Autodesk Fusion 360 part; units mm, degrees
(part 6 of 9)
sketch "草图17 (8)" plane through (593, 0, 0) normal (1, 0, 0) x (0, 0, -1) in component "R1_DrainPan"
  line L0 (-24.9649, 136.9) -> (-24.6782, 141)
  line L1 (-24.6782, 141) -> (-41, 141)
  line L2 (-41, 141) -> (-41, 136.9)
  line L3 (-41, 136.9) -> (-24.9649, 136.9)
  dimension "d2420" = 24.9649
  dimension "d2421" = 136.9
  dimension "d2422" = 24.6782
  dimension "d2423" = 141
  dimension "d2424" = 41
  constraint horizontal L1
  constraint vertical L2
  constraint horizontal L3
  measures "d2420" horizontal distance of origin L0.start
  measures "d2421" vertical distance of origin L0.start
  measures "d2422" horizontal distance of origin L0.end
  measures "d2423" vertical distance of origin L0.end
  measures "d2424" horizontal distance of origin L1.end
extrude "R02 full width open front''" cut sketch "草图17 (8)" along normal blind 128 bodies 13 in component "R1_DrainPan"
ref_plane "工作平面14" through (0, 0, 36) normal (0, 0, 1) x (1, 0, 0) in component "R1_RemovableGrate"
sketch "草图14 (13)" plane through (0, 0, 36) normal (0, 0, 1) x (1, 0, 0) in component "R1_RemovableGrate"
  line L0 (592.7, 59.7) -> (595.3, 59.7)
  line L1 (595.3, 59.7) -> (595.3, 65.3)
  line L2 (595.3, 65.3) -> (592.7, 65.3)
  line L3 (592.7, 65.3) -> (592.7, 59.7)
  dimension "d2430" = 59.7
  dimension "d2431" = 2.6
  dimension "d2432" = 5.6
  constraint horizontal L0
  constraint vertical L1
  constraint horizontal L2
  constraint vertical L3
  measures "d2430" vertical distance of origin L0.start
  measures "d2431" horizontal distance of L0.start L0.end
  measures "d2432" vertical distance of L0.end L1.end
extrude "R02 side locating notch 0''" cut sketch "草图14 (13)" along normal blind 4 bodies 14 in component "R1_RemovableGrate"
ref_plane "工作平面18" through (0, 0, 20) normal (0, 0, 1) x (1, 0, 0) in component "R1_DrainPan"
sketch "草图18 (4)" plane through (0, 0, 20) normal (0, 0, 1) x (1, 0, 0) in component "R1_DrainPan"
  line L0 (593, 60) -> (595, 60)
  line L1 (595, 60) -> (595, 65)
  line L2 (595, 65) -> (593, 65)
  line L3 (593, 65) -> (593, 60)
  dimension "d2438" = 60
  dimension "d2439" = 2
  dimension "d2440" = 5
  constraint horizontal L0
  constraint vertical L1
  constraint horizontal L2
  constraint vertical L3
  measures "d2438" vertical distance of origin L0.start
  measures "d2439" horizontal distance of L0.start L0.end
  measures "d2440" vertical distance of L0.end L1.end
extrude "R02 side locating key 0''" add sketch "草图18 (4)" along normal blind 20 bodies 13 in component "R1_DrainPan"
ref_plane "工作平面15" through (0, 0, 36) normal (0, 0, 1) x (1, 0, 0) in component "R1_RemovableGrate"
sketch "草图15 (13)" plane through (0, 0, 36) normal (0, 0, 1) x (1, 0, 0) in component "R1_RemovableGrate"
  line L0 (718.7, 59.7) -> (721.3, 59.7)
  line L1 (721.3, 59.7) -> (721.3, 65.3)
  line L2 (721.3, 65.3) -> (718.7, 65.3)
  line L3 (718.7, 65.3) -> (718.7, 59.7)
  dimension "d2445" = 718.7
  dimension "d2446" = 59.7
  dimension "d2447" = 2.6
  dimension "d2448" = 5.6
  constraint horizontal L0
  constraint vertical L1
  constraint horizontal L2
  constraint vertical L3
  measures "d2445" horizontal distance of origin L0.start
  measures "d2446" vertical distance of origin L0.start
  measures "d2447" horizontal distance of L0.start L0.end
  measures "d2448" vertical distance of L0.end L1.end
extrude "R02 side locating notch 1''" cut sketch "草图15 (13)" along normal blind 4 bodies 14 in component "R1_RemovableGrate"
ref_plane "工作平面19" through (0, 0, 20) normal (0, 0, 1) x (1, 0, 0) in component "R1_DrainPan"
sketch "草图19 (4)" plane through (0, 0, 20) normal (0, 0, 1) x (1, 0, 0) in component "R1_DrainPan"
  line L0 (719, 60) -> (721, 60)
  line L1 (721, 60) -> (721, 65)
  line L2 (721, 65) -> (719, 65)
  line L3 (719, 65) -> (719, 60)
  dimension "d2453" = 719
  dimension "d2454" = 60
  dimension "d2455" = 2
  dimension "d2456" = 5
  constraint horizontal L0
  constraint vertical L1
  constraint horizontal L2
  constraint vertical L3
  measures "d2453" horizontal distance of origin L0.start
  measures "d2454" vertical distance of origin L0.start
  measures "d2455" horizontal distance of L0.start L0.end
  measures "d2456" vertical distance of L0.end L1.end
extrude "R02 side locating key 1''" add sketch "草图19 (4)" along normal blind 20 bodies 13 in component "R1_DrainPan"
ref_plane "工作平面16" through (0, 0, 19.8) normal (0, 0, 1) x (1, 0, 0) in component "R2_DrainPan"
sketch "草图16 (9)" plane through (0, 0, 19.8) normal (0, 0, 1) x (1, 0, 0) in component "R2_DrainPan"
  line L0 (725, 140) -> (861, 140)
  line L1 (861, 140) -> (861, 167)
  line L2 (861, 167) -> (725, 167)
  line L3 (725, 167) -> (725, 140)
  dimension "d2461" = 725
  dimension "d2463" = 136
  dimension "d2464" = 27
  constraint horizontal L0
  constraint vertical L1
  constraint horizontal L2
  constraint vertical L3
  measures "d2461" horizontal distance of origin L0.start
  measures "d2463" horizontal distance of L0.start L0.end
  measures "d2464" vertical distance of L0.end L1.end
extrude "R02 remove projecting spout'''" cut sketch "草图16 (9)" along normal blind 20.4 bodies 19 in component "R2_DrainPan"
ref_plane "工作平面17" through (729, 0, 0) normal (1, 0, 0) x (0, 1, 0) in component "R2_DrainPan"
sketch "草图17 (9)" plane through (729, 0, 0) normal (1, 0, 0) x (0, 0, -1) in component "R2_DrainPan"
  line L0 (-24.9649, 136.9) -> (-24.6782, 141)
  line L1 (-24.6782, 141) -> (-41, 141)
  line L2 (-41, 141) -> (-41, 136.9)
  line L3 (-41, 136.9) -> (-24.9649, 136.9)
  dimension "d2469" = 24.9649
  dimension "d2470" = 136.9
  dimension "d2471" = 24.6782
  dimension "d2472" = 141
  dimension "d2473" = 41
  constraint horizontal L1
  constraint vertical L2
  constraint horizontal L3
  measures "d2469" horizontal distance of origin L0.start
  measures "d2470" vertical distance of origin L0.start
  measures "d2471" horizontal distance of origin L0.end
  measures "d2472" vertical distance of origin L0.end
  measures "d2473" horizontal distance of origin L1.end
extrude "R02 full width open front'''" cut sketch "草图17 (9)" along normal blind 128 bodies 19 in component "R2_DrainPan"
ref_plane "工作平面14" through (0, 0, 36) normal (0, 0, 1) x (1, 0, 0) in component "R2_RemovableGrate"
sketch "草图14 (14)" plane through (0, 0, 36) normal (0, 0, 1) x (1, 0, 0) in component "R2_RemovableGrate"
  line L0 (728.7, 59.7) -> (731.3, 59.7)
  line L1 (731.3, 59.7) -> (731.3, 65.3)
  line L2 (731.3, 65.3) -> (728.7, 65.3)
  line L3 (728.7, 65.3) -> (728.7, 59.7)
  dimension "d2478" = 728.7
  dimension "d2479" = 59.7
  dimension "d2480" = 2.6
  dimension "d2481" = 5.6
  constraint horizontal L0
  constraint vertical L1
  constraint horizontal L2
  constraint vertical L3
  measures "d2478" horizontal distance of origin L0.start
  measures "d2479" vertical distance of origin L0.start
  measures "d2480" horizontal distance of L0.start L0.end
  measures "d2481" vertical distance of L0.end L1.end
extrude "R02 side locating notch 0'''" cut sketch "草图14 (14)" along normal blind 4 bodies 20 in component "R2_RemovableGrate"
ref_plane "工作平面18" through (0, 0, 20) normal (0, 0, 1) x (1, 0, 0) in component "R2_DrainPan"
sketch "草图18 (5)" plane through (0, 0, 20) normal (0, 0, 1) x (1, 0, 0) in component "R2_DrainPan"
  line L0 (729, 60) -> (731, 60)
  line L1 (731, 60) -> (731, 65)
  line L2 (731, 65) -> (729, 65)
  line L3 (729, 65) -> (729, 60)
  dimension "d2486" = 729
  dimension "d2487" = 60
  dimension "d2488" = 2
  dimension "d2489" = 5
  constraint horizontal L0
  constraint vertical L1
  constraint horizontal L2
  constraint vertical L3
  measures "d2486" horizontal distance of origin L0.start
  measures "d2487" vertical distance of origin L0.start
  measures "d2488" horizontal distance of L0.start L0.end
  measures "d2489" vertical distance of L0.end L1.end
extrude "R02 side locating key 0'''" add sketch "草图18 (5)" along normal blind 20 bodies 19 in component "R2_DrainPan"
ref_plane "工作平面15" through (0, 0, 36) normal (0, 0, 1) x (1, 0, 0) in component "R2_RemovableGrate"
sketch "草图15 (14)" plane through (0, 0, 36) normal (0, 0, 1) x (1, 0, 0) in component "R2_RemovableGrate"
  line L0 (854.7, 59.7) -> (857.3, 59.7)
  line L1 (857.3, 59.7) -> (857.3, 65.3)
  line L2 (857.3, 65.3) -> (854.7, 65.3)
  line L3 (854.7, 65.3) -> (854.7, 59.7)
  dimension "d2494" = 854.7
  dimension "d2495" = 59.7
  dimension "d2496" = 2.6
  dimension "d2497" = 5.6
  constraint horizontal L0
  constraint vertical L1
  constraint horizontal L2
  constraint vertical L3
  measures "d2494" horizontal distance of origin L0.start
  measures "d2495" vertical distance of origin L0.start
  measures "d2496" horizontal distance of L0.start L0.end
  measures "d2497" vertical distance of L0.end L1.end
extrude "R02 side locating notch 1'''" cut sketch "草图15 (14)" along normal blind 4 bodies 20 in component "R2_RemovableGrate"
ref_plane "工作平面19" through (0, 0, 20) normal (0, 0, 1) x (1, 0, 0) in component "R2_DrainPan"
sketch "草图19 (5)" plane through (0, 0, 20) normal (0, 0, 1) x (1, 0, 0) in component "R2_DrainPan"
  line L0 (855, 60) -> (857, 60)
  line L1 (857, 60) -> (857, 65)
  line L2 (857, 65) -> (855, 65)
  line L3 (855, 65) -> (855, 60)
  dimension "d2502" = 855
  dimension "d2503" = 60
  dimension "d2504" = 2
  dimension "d2505" = 5
  constraint horizontal L0
  constraint vertical L1
  constraint horizontal L2
  constraint vertical L3
  measures "d2502" horizontal distance of origin L0.start
  measures "d2503" vertical distance of origin L0.start
  measures "d2504" horizontal distance of L0.start L0.end
  measures "d2505" vertical distance of L0.end L1.end
extrude "R02 side locating key 1'''" add sketch "草图19 (5)" along normal blind 20 bodies 19 in component "R2_DrainPan"
ref_plane "工作平面16" through (0, 0, 19.8) normal (0, 0, 1) x (1, 0, 0) in component "LS_DrainPan"
sketch "草图16 (10)" plane through (0, 0, 19.8) normal (0, 0, 1) x (1, 0, 0) in component "LS_DrainPan"
  line L0 (170, 141) -> (197, 141)
  line L1 (197, 141) -> (197, 323)
  line L2 (197, 323) -> (170, 323)
  line L3 (170, 323) -> (170, 141)
  dimension "d2511" = 141
  dimension "d2512" = 27
  dimension "d2513" = 182
  constraint horizontal L0
  constraint vertical L1
  constraint horizontal L2
  constraint vertical L3
  measures "d2511" vertical distance of origin L0.start
  measures "d2512" horizontal distance of L0.start L0.end
  measures "d2513" vertical distance of L0.end L1.end
extrude "R02 remove projecting spout''''" cut sketch "草图16 (10)" along normal blind 20.4 bodies 25 in component "LS_DrainPan"
ref_plane "工作平面17" through (0, 319, 0) normal (0, 1, 0) x (0, 0, 1) in component "LS_DrainPan"
sketch "草图17 (10)" plane through (0, 319, 0) normal (0, 1, 0) x (1, 0, 0) in component "LS_DrainPan"
  line L0 (166.9, -24.9649) -> (171, -24.6782)
  line L1 (171, -24.6782) -> (171, -41)
  line L2 (171, -41) -> (166.9, -41)
  line L3 (166.9, -41) -> (166.9, -24.9649)
  dimension "d2518" = 166.9
  dimension "d2519" = 24.9649
  dimension "d2520" = 171
  dimension "d2521" = 24.6782
  dimension "d2522" = 41
  constraint vertical L1
  constraint horizontal L2
  constraint vertical L3
  measures "d2518" horizontal distance of origin L0.start
  measures "d2519" vertical distance of origin L0.start
  measures "d2520" horizontal distance of origin L0.end
  measures "d2521" vertical distance of origin L0.end
  measures "d2522" vertical distance of origin L1.end
extrude "R02 full width open front''''" cut sketch "草图17 (10)" against normal blind 174 bodies 25 in component "LS_DrainPan"
ref_plane "工作平面18" through (0, 0, 36) normal (0, 0, 1) x (1, 0, 0) in component "LS_RemovableGrate"
sketch "草图18 (6)" plane through (0, 0, 36) normal (0, 0, 1) x (1, 0, 0) in component "LS_RemovableGrate"
  line L0 (59.7, 316.7) -> (65.3, 316.7)
  line L1 (65.3, 316.7) -> (65.3, 319.3)
  line L2 (65.3, 319.3) -> (59.7, 319.3)
  line L3 (59.7, 319.3) -> (59.7, 316.7)
  dimension "d2527" = 59.7
  dimension "d2528" = 316.7
  dimension "d2529" = 5.6
  dimension "d2530" = 2.6
  constraint horizontal L0
  constraint vertical L1
  constraint horizontal L2
  constraint vertical L3
  measures "d2527" horizontal distance of origin L0.start
  measures "d2528" vertical distance of origin L0.start
  measures "d2529" horizontal distance of L0.start L0.end
  measures "d2530" vertical distance of L0.end L1.end
extrude "R02 side locating notch 0''''" cut sketch "草图18 (6)" along normal blind 4 bodies 26 in component "LS_RemovableGrate"
ref_plane "工作平面18" through (0, 0, 20) normal (0, 0, 1) x (1, 0, 0) in component "LS_DrainPan"
sketch "草图18 (7)" plane through (0, 0, 20) normal (0, 0, 1) x (1, 0, 0) in component "LS_DrainPan"
  line L0 (60, 317) -> (65, 317)
  line L1 (65, 317) -> (65, 319)
  line L2 (65, 319) -> (60, 319)
  line L3 (60, 319) -> (60, 317)
  dimension "d2535" = 60
  dimension "d2536" = 317
  dimension "d2537" = 5
  dimension "d2538" = 2
  constraint horizontal L0
  constraint vertical L1
  constraint horizontal L2
  constraint vertical L3
  measures "d2535" horizontal distance of origin L0.start
  measures "d2536" vertical distance of origin L0.start
  measures "d2537" horizontal distance of L0.start L0.end
  measures "d2538" vertical distance of L0.end L1.end
extrude "R02 side locating key 0''''" add sketch "草图18 (7)" along normal blind 20 bodies 25 in component "LS_DrainPan"
ref_plane "工作平面19" through (0, 0, 36) normal (0, 0, 1) x (1, 0, 0) in component "LS_RemovableGrate"
sketch "草图19 (6)" plane through (0, 0, 36) normal (0, 0, 1) x (1, 0, 0) in component "LS_RemovableGrate"
  line L0 (59.7, 144.7) -> (65.3, 144.7)
  line L1 (65.3, 144.7) -> (65.3, 147.3)
  line L2 (65.3, 147.3) -> (59.7, 147.3)
  line L3 (59.7, 147.3) -> (59.7, 144.7)
  dimension "d2543" = 59.7
  dimension "d2544" = 144.7
  dimension "d2545" = 5.6
  dimension "d2546" = 2.6
  constraint horizontal L0
  constraint vertical L1
  constraint horizontal L2
  constraint vertical L3
  measures "d2543" horizontal distance of origin L0.start
  measures "d2544" vertical distance of origin L0.start
  measures "d2545" horizontal distance of L0.start L0.end
  measures "d2546" vertical distance of L0.end L1.end
extrude "R02 side locating notch 1''''" cut sketch "草图19 (6)" along normal blind 4 bodies 26 in component "LS_RemovableGrate"
ref_plane "工作平面19" through (0, 0, 20) normal (0, 0, 1) x (1, 0, 0) in component "LS_DrainPan"
sketch "草图19 (7)" plane through (0, 0, 20) normal (0, 0, 1) x (1, 0, 0) in component "LS_DrainPan"
  line L0 (60, 145) -> (65, 145)
  line L1 (65, 145) -> (65, 147)
  line L2 (65, 147) -> (60, 147)
  line L3 (60, 147) -> (60, 145)
  dimension "d2551" = 60
  dimension "d2552" = 145
  dimension "d2553" = 5
  dimension "d2554" = 2
  constraint horizontal L0
  constraint vertical L1
  constraint horizontal L2
  constraint vertical L3
  measures "d2551" horizontal distance of origin L0.start
  measures "d2552" vertical distance of origin L0.start
  measures "d2553" horizontal distance of L0.start L0.end
  measures "d2554" vertical distance of L0.end L1.end
extrude "R02 side locating key 1''''" add sketch "草图19 (7)" along normal blind 20 bodies 25 in component "LS_DrainPan"
ref_plane "工作平面16" through (0, 0, 19.8) normal (0, 0, 1) x (1, 0, 0) in component "RS_DrainPan"
sketch "草图16 (11)" plane through (0, 0, 19.8) normal (0, 0, 1) x (1, 0, 0) in component "RS_DrainPan"
  line L0 (743, 141) -> (770, 141)
  line L1 (770, 141) -> (770, 323)
  line L2 (770, 323) -> (743, 323)
  line L3 (743, 323) -> (743, 141)
  dimension "d2559" = 743
  dimension "d2560" = 141
  dimension "d2561" = 27
  dimension "d2562" = 182
  constraint horizontal L0
  constraint vertical L1
  constraint horizontal L2
  constraint vertical L3
  measures "d2559" horizontal distance of origin L0.start
  measures "d2560" vertical distance of origin L0.start
  measures "d2561" horizontal distance of L0.start L0.end
  measures "d2562" vertical distance of L0.end L1.end
extrude "R02 remove projecting spout'''''" cut sketch "草图16 (11)" along normal blind 20.4 bodies 31 in component "RS_DrainPan"
ref_plane "工作平面17" through (0, 145, 0) normal (0, 1, 0) x (0, 0, 1) in component "RS_DrainPan"
sketch "草图17 (11)" plane through (0, 145, 0) normal (0, 1, 0) x (1, 0, 0) in component "RS_DrainPan"
  line L0 (773.1, -24.9649) -> (769, -24.6782)
  line L1 (769, -24.6782) -> (769, -41)
  line L2 (769, -41) -> (773.1, -41)
  line L3 (773.1, -41) -> (773.1, -24.9649)
  dimension "d2567" = 773.1
  dimension "d2568" = 24.9649
  dimension "d2569" = 769
  dimension "d2570" = 24.6782
  dimension "d2571" = 41
  constraint vertical L1
  constraint horizontal L2
  constraint vertical L3
  measures "d2567" horizontal distance of origin L0.start
  measures "d2568" vertical distance of origin L0.start
  measures "d2569" horizontal distance of origin L0.end
  measures "d2570" vertical distance of origin L0.end
  measures "d2571" vertical distance of origin L1.end
extrude "R02 full width open front'''''" cut sketch "草图17 (11)" along normal blind 174 bodies 31 in component "RS_DrainPan"
ref_plane "工作平面18" through (0, 0, 36) normal (0, 0, 1) x (1, 0, 0) in component "RS_RemovableGrate"
sketch "草图18 (8)" plane through (0, 0, 36) normal (0, 0, 1) x (1, 0, 0) in component "RS_RemovableGrate"
  line L0 (844.7, 144.7) -> (850.3, 144.7)
  line L1 (850.3, 144.7) -> (850.3, 147.3)
  line L2 (850.3, 147.3) -> (844.7, 147.3)
  line L3 (844.7, 147.3) -> (844.7, 144.7)
  dimension "d2576" = 844.7
  dimension "d2578" = 5.6
  dimension "d2579" = 2.6
  constraint horizontal L0
  constraint vertical L1
  constraint horizontal L2
  constraint vertical L3
  measures "d2576" horizontal distance of origin L0.start
  measures "d2578" horizontal distance of L0.start L0.end
  measures "d2579" vertical distance of L0.end L1.end
extrude "R02 side locating notch 0'''''" cut sketch "草图18 (8)" along normal blind 4 bodies 32 in component "RS_RemovableGrate"
ref_plane "工作平面18" through (0, 0, 20) normal (0, 0, 1) x (1, 0, 0) in component "RS_DrainPan"
sketch "草图18 (9)" plane through (0, 0, 20) normal (0, 0, 1) x (1, 0, 0) in component "RS_DrainPan"
  line L0 (845, 145) -> (850, 145)
  line L1 (850, 145) -> (850, 147)
  line L2 (850, 147) -> (845, 147)
  line L3 (845, 147) -> (845, 145)
  dimension "d2584" = 845
  dimension "d2586" = 5
  dimension "d2587" = 2
  constraint horizontal L0
  constraint vertical L1
  constraint horizontal L2
  constraint vertical L3
  measures "d2584" horizontal distance of origin L0.start
  measures "d2586" horizontal distance of L0.start L0.end
  measures "d2587" vertical distance of L0.end L1.end
extrude "R02 side locating key 0'''''" add sketch "草图18 (9)" along normal blind 20 bodies 31 in component "RS_DrainPan"
ref_plane "工作平面19" through (0, 0, 36) normal (0, 0, 1) x (1, 0, 0) in component "RS_RemovableGrate"
sketch "草图19 (8)" plane through (0, 0, 36) normal (0, 0, 1) x (1, 0, 0) in component "RS_RemovableGrate"
  line L0 (844.7, 316.7) -> (850.3, 316.7)
  line L1 (850.3, 316.7) -> (850.3, 319.3)
  line L2 (850.3, 319.3) -> (844.7, 319.3)
  line L3 (844.7, 319.3) -> (844.7, 316.7)
  dimension "d2592" = 844.7
  dimension "d2593" = 316.7
  dimension "d2594" = 5.6
  dimension "d2595" = 2.6
  constraint horizontal L0
  constraint vertical L1
  constraint horizontal L2
  constraint vertical L3
  measures "d2592" horizontal distance of origin L0.start
  measures "d2593" vertical distance of origin L0.start
  measures "d2594" horizontal distance of L0.start L0.end
  measures "d2595" vertical distance of L0.end L1.end
extrude "R02 side locating notch 1'''''" cut sketch "草图19 (8)" along normal blind 4 bodies 32 in component "RS_RemovableGrate"
ref_plane "工作平面19" through (0, 0, 20) normal (0, 0, 1) x (1, 0, 0) in component "RS_DrainPan"
sketch "草图19 (9)" plane through (0, 0, 20) normal (0, 0, 1) x (1, 0, 0) in component "RS_DrainPan"
  line L0 (845, 317) -> (850, 317)
  line L1 (850, 317) -> (850, 319)
  line L2 (850, 319) -> (845, 319)
  line L3 (845, 319) -> (845, 317)
  dimension "d2600" = 845
  dimension "d2601" = 317
  dimension "d2602" = 5
  dimension "d2603" = 2
  constraint horizontal L0
  constraint vertical L1
  constraint horizontal L2
  constraint vertical L3
  measures "d2600" horizontal distance of origin L0.start
  measures "d2601" vertical distance of origin L0.start
  measures "d2602" horizontal distance of L0.start L0.end
  measures "d2603" vertical distance of L0.end L1.end
extrude "R02 side locating key 1'''''" add sketch "草图19 (9)" along normal blind 20 bodies 31 in component "RS_DrainPan"
ref_plane "工作平面16" through (0, 0, 124.8) normal (0, 0, 1) x (1, 0, 0) in component "UP_DrainPan"
sketch "草图16 (12)" plane through (0, 0, 124.8) normal (0, 0, 1) x (1, 0, 0) in component "UP_DrainPan"
  line L0 (49, 140) -> (231, 140)
  line L1 (231, 140) -> (231, 167)
  line L2 (231, 167) -> (49, 167)
  line L3 (49, 167) -> (49, 140)
  dimension "d2608" = 49
  dimension "d2610" = 182
  dimension "d2611" = 27
  constraint horizontal L0
  constraint vertical L1
  constraint horizontal L2
  constraint vertical L3
  measures "d2608" horizontal distance of origin L0.start
  measures "d2610" horizontal distance of L0.start L0.end
  measures "d2611" vertical distance of L0.end L1.end
extrude "R02 remove projecting spout''''''" cut sketch "草图16 (12)" along normal blind 20.4 bodies 37 in component "UP_DrainPan"
ref_plane "工作平面17" through (53, 0, 0) normal (1, 0, 0) x (0, 1, 0) in component "UP_DrainPan"
sketch "草图17 (12)" plane through (53, 0, 0) normal (1, 0, 0) x (0, 0, -1) in component "UP_DrainPan"
  line L0 (-129.9649, 136.9) -> (-129.6782, 141)
  line L1 (-129.6782, 141) -> (-146, 141)
  line L2 (-146, 141) -> (-146, 136.9)
  line L3 (-146, 136.9) -> (-129.9649, 136.9)
  dimension "d2616" = 129.9649
  dimension "d2617" = 136.9
  dimension "d2618" = 129.6782
  dimension "d2619" = 141
  dimension "d2620" = 146
  constraint horizontal L1
  constraint vertical L2
  constraint horizontal L3
  measures "d2616" horizontal distance of origin L0.start
  measures "d2617" vertical distance of origin L0.start
  measures "d2618" horizontal distance of origin L0.end
  measures "d2619" vertical distance of origin L0.end
  measures "d2620" horizontal distance of origin L1.end
extrude "R02 full width open front''''''" cut sketch "草图17 (12)" along normal blind 174 bodies 37 in component "UP_DrainPan"
ref_plane "工作平面18" through (0, 0, 141) normal (0, 0, 1) x (1, 0, 0) in component "UP_RemovableGrate"
sketch "草图18 (10)" plane through (0, 0, 141) normal (0, 0, 1) x (1, 0, 0) in component "UP_RemovableGrate"
  line L0 (52.7, 62.7) -> (55.3, 62.7)
  line L1 (55.3, 62.7) -> (55.3, 68.3)
  line L2 (55.3, 68.3) -> (52.7, 68.3)
  line L3 (52.7, 68.3) -> (52.7, 62.7)
  dimension "d2626" = 62.7
  dimension "d2627" = 2.6
  dimension "d2628" = 5.6
  constraint horizontal L0
  constraint vertical L1
  constraint horizontal L2
  constraint vertical L3
  measures "d2626" vertical distance of origin L0.start
  measures "d2627" horizontal distance of L0.start L0.end
  measures "d2628" vertical distance of L0.end L1.end
extrude "R02 side locating notch 0''''''" cut sketch "草图18 (10)" along normal blind 4 bodies 38 in component "UP_RemovableGrate"
ref_plane "工作平面18" through (0, 0, 125) normal (0, 0, 1) x (1, 0, 0) in component "UP_DrainPan"
sketch "草图18 (11)" plane through (0, 0, 125) normal (0, 0, 1) x (1, 0, 0) in component "UP_DrainPan"
  line L0 (53, 63) -> (55, 63)
  line L1 (55, 63) -> (55, 68)
  line L2 (55, 68) -> (53, 68)
  line L3 (53, 68) -> (53, 63)
  dimension "d2634" = 63
  dimension "d2635" = 2
  dimension "d2636" = 5
  constraint horizontal L0
  constraint vertical L1
  constraint horizontal L2
  constraint vertical L3
  measures "d2634" vertical distance of origin L0.start
  measures "d2635" horizontal distance of L0.start L0.end
  measures "d2636" vertical distance of L0.end L1.end
extrude "R02 side locating key 0''''''" add sketch "草图18 (11)" along normal blind 20 bodies 37 in component "UP_DrainPan"
ref_plane "工作平面19" through (0, 0, 141) normal (0, 0, 1) x (1, 0, 0) in component "UP_RemovableGrate"
sketch "草图19 (10)" plane through (0, 0, 141) normal (0, 0, 1) x (1, 0, 0) in component "UP_RemovableGrate"
  line L0 (224.7, 62.7) -> (227.3, 62.7)
  line L1 (227.3, 62.7) -> (227.3, 68.3)
  line L2 (227.3, 68.3) -> (224.7, 68.3)
  line L3 (224.7, 68.3) -> (224.7, 62.7)
  dimension "d2641" = 224.7
  dimension "d2642" = 62.7
  dimension "d2643" = 2.6
  dimension "d2644" = 5.6
  constraint horizontal L0
  constraint vertical L1
  constraint horizontal L2
  constraint vertical L3
  measures "d2641" horizontal distance of origin L0.start
  measures "d2642" vertical distance of origin L0.start
  measures "d2643" horizontal distance of L0.start L0.end
  measures "d2644" vertical distance of L0.end L1.end
extrude "R02 side locating notch 1''''''" cut sketch "草图19 (10)" along normal blind 4 bodies 38 in component "UP_RemovableGrate"
ref_plane "工作平面19" through (0, 0, 125) normal (0, 0, 1) x (1, 0, 0) in component "UP_DrainPan"
sketch "草图19 (11)" plane through (0, 0, 125) normal (0, 0, 1) x (1, 0, 0) in component "UP_DrainPan"
  line L0 (225, 63) -> (227, 63)
  line L1 (227, 63) -> (227, 68)
  line L2 (227, 68) -> (225, 68)
  line L3 (225, 68) -> (225, 63)
  dimension "d2649" = 225
  dimension "d2650" = 63
  dimension "d2651" = 2
  dimension "d2652" = 5
  constraint horizontal L0
  constraint vertical L1
  constraint horizontal L2
  constraint vertical L3
  measures "d2649" horizontal distance of origin L0.start
  measures "d2650" vertical distance of origin L0.start
  measures "d2651" horizontal distance of L0.start L0.end
  measures "d2652" vertical distance of L0.end L1.end
extrude "R02 side locating key 1''''''" add sketch "草图19 (11)" along normal blind 20 bodies 37 in component "UP_DrainPan"
component "L1_DrainPan" placed x (1, 0, 0) y (0, 1, 0) z (0, 0, 1) at (0, 0, 0)
component "L1_RemovableGrate" placed x (1, 0, 0) y (0, 1, 0) z (0, 0, 1) at (0, 0, 0)
component "L1_Foot_00" placed x (1, 0, 0) y (0, 1, 0) z (0, 0, 1) at (0, 0, 0)
component "L1_Foot_01" placed x (1, 0, 0) y (0, 1, 0) z (0, 0, 1) at (0, 0, 0)
component "L1_Foot_10" placed x (1, 0, 0) y (0, 1, 0) z (0, 0, 1) at (0, 0, 0)
component "L1_Foot_11" placed x (1, 0, 0) y (0, 1, 0) z (0, 0, 1) at (0, 0, 0)
component "L2_DrainPan" placed x (1, 0, 0) y (0, 1, 0) z (0, 0, 1) at (0, 0, 0)
component "L2_RemovableGrate" placed x (1, 0, 0) y (0, 1, 0) z (0, 0, 1) at (0, 0, 0)
component "L2_Foot_00" placed x (1, 0, 0) y (0, 1, 0) z (0, 0, 1) at (0, 0, 0)
component "L2_Foot_01" placed x (1, 0, 0) y (0, 1, 0) z (0, 0, 1) at (0, 0, 0)
component "L2_Foot_10" placed x (1, 0, 0) y (0, 1, 0) z (0, 0, 1) at (0, 0, 0)
component "L2_Foot_11" placed x (1, 0, 0) y (0, 1, 0) z (0, 0, 1) at (0, 0, 0)
component "R1_DrainPan" placed x (1, 0, 0) y (0, 1, 0) z (0, 0, 1) at (0, 0, 0)
component "R1_RemovableGrate" placed x (1, 0, 0) y (0, 1, 0) z (0, 0, 1) at (0, 0, 0)
component "R1_Foot_00" placed x (1, 0, 0) y (0, 1, 0) z (0, 0, 1) at (0, 0, 0)
component "R1_Foot_01" placed x (1, 0, 0) y (0, 1, 0) z (0, 0, 1) at (0, 0, 0)
component "R1_Foot_10" placed x (1, 0, 0) y (0, 1, 0) z (0, 0, 1) at (0, 0, 0)
component "R1_Foot_11" placed x (1, 0, 0) y (0, 1, 0) z (0, 0, 1) at (0, 0, 0)
component "R2_DrainPan" placed x (1, 0, 0) y (0, 1, 0) z (0, 0, 1) at (0, 0, 0)
component "R2_RemovableGrate" placed x (1, 0, 0) y (0, 1, 0) z (0, 0, 1) at (0, 0, 0)
component "R2_Foot_00" placed x (1, 0, 0) y (0, 1, 0) z (0, 0, 1) at (0, 0, 0)
component "R2_Foot_01" placed x (1, 0, 0) y (0, 1, 0) z (0, 0, 1) at (0, 0, 0)
component "R2_Foot_10" placed x (1, 0, 0) y (0, 1, 0) z (0, 0, 1) at (0, 0, 0)
component "R2_Foot_11" placed x (1, 0, 0) y (0, 1, 0) z (0, 0, 1) at (0, 0, 0)
component "LS_DrainPan" placed x (1, 0, 0) y (0, 1, 0) z (0, 0, 1) at (0, 0, 0)
component "LS_RemovableGrate" placed x (1, 0, 0) y (0, 1, 0) z (0, 0, 1) at (0, 0, 0)
component "LS_Foot_00" placed x (1, 0, 0) y (0, 1, 0) z (0, 0, 1) at (0, 0, 0)
component "LS_Foot_01" placed x (1, 0, 0) y (0, 1, 0) z (0, 0, 1) at (0, 0, 0)
component "LS_Foot_10" placed x (1, 0, 0) y (0, 1, 0) z (0, 0, 1) at (0, 0, 0)
component "LS_Foot_11" placed x (1, 0, 0) y (0, 1, 0) z (0, 0, 1) at (0, 0, 0)
component "RS_DrainPan" placed x (1, 0, 0) y (0, 1, 0) z (0, 0, 1) at (0, 0, 0)
component "RS_RemovableGrate" placed x (1, 0, 0) y (0, 1, 0) z (0, 0, 1) at (0, 0, 0)
component "RS_Foot_00" placed x (1, 0, 0) y (0, 1, 0) z (0, 0, 1) at (0, 0, 0)
component "RS_Foot_01" placed x (1, 0, 0) y (0, 1, 0) z (0, 0, 1) at (0, 0, 0)
component "RS_Foot_10" placed x (1, 0, 0) y (0, 1, 0) z (0, 0, 1) at (0, 0, 0)
component "RS_Foot_11" placed x (1, 0, 0) y (0, 1, 0) z (0, 0, 1) at (0, 0, 0)
component "UP_DrainPan" placed x (1, 0, 0) y (0, 1, 0) z (0, 0, 1) at (0, 0, 0)
component "UP_RemovableGrate" placed x (1, 0, 0) y (0, 1, 0) z (0, 0, 1) at (0, 0, 0)
component "Tower_SideFrame_1" placed x (1, 0, 0) y (0, 1, 0) z (0, 0, 1) at (0, 0, 0)
component "Tower_SideFrame_2" placed x (1, 0, 0) y (0, 1, 0) z (0, 0, 1) at (0, 0, 0)
component "FIT_Tight" placed x (1, 0, 0) y (0, 1, 0) z (0, 0, 1) at (0, 0, 0)
component "FIT_Nominal" placed x (1, 0, 0) y (0, 1, 0) z (0, 0, 1) at (0, 0, 0)
component "FIT_Loose" placed x (1, 0, 0) y (0, 1, 0) z (0, 0, 1) at (0, 0, 0)
equation "LeftAvailable = 400 mm" comment "User approximate dimension: left of faucet"
equation "RightAvailable = 300 mm" comment "User approximate dimension: right of faucet"
equation "RearAvailable = 100 mm" comment "User approximate rear strip depth"
equation "LeftSideAvailable = 130 mm" comment "User approximate left strip width"
equation "MirrorClearance = 300 mm" comment "User approximate countertop to mirror cabinet"
equation "RightSideAvailable = 100 mm" comment "ASSUMPTION: awaiting measurement"
equation "LeftReach = 180 mm" comment "ASSUMPTION: forward side extension beyond rear rack"
equation "RightReach = 180 mm" comment "ASSUMPTION: forward side extension beyond rear rack"
equation "FaucetGap = 160 mm" comment "ASSUMPTION: faucet and lever clearance, awaiting measurement"
equation "LeftRun = LeftAvailable - 20 mm" comment "Design clearance allowance; check on site"
equation "RightRun = RightAvailable - 30 mm" comment "Design clearance allowance; check lever"
equation "Depth = RearAvailable - 10 mm" comment "Rear standing module depth"
equation "LeftSideDepth = LeftSideAvailable - 10 mm" comment "Left side module depth"
equation "RightSideDepth = RightSideAvailable - 10 mm" comment "Right side module depth, provisional"
equation "ModuleGap = 2 mm" comment "Open cleaning / assembly seam, not watertight"
equation "TowerWidth = 180 mm" comment "Local upper tier only"
equation "TowerFrame = 8 mm" comment "Side portal frame thickness"
equation "TowerClearance = 2 mm" comment "Clearance from lower tray to side frames"
equation "FootHeight = 20 mm" comment "Clear gap below pan"
equation "PanHeight = 20 mm" comment "Pan rim above underside"
equation "FloorMin = 3 mm" comment "Minimum pan floor at outlet"
equation "Wall = 3 mm" comment "Pan walls"
equation "DrainSlope = 4 deg" comment "Initial design slope; verify with water test"
equation "DeckThick = 4 mm" comment "Removable horizontal grate thickness"
equation "DeckClearance = 0.3 mm" comment "Per-side clearance; fit coupon required"
equation "RimBorder = 7 mm" comment "Solid grate border"
equation "SlotWidth = 4 mm" comment "Open slat gaps"
equation "SlotPitch = 10 mm" comment "Initial grate slot spacing"
equation "DrainWidth = 28 mm" comment "R01 construction history only: R02 opens the entire front between side walls"
equation "DrainExtension = 25 mm" comment "R01 construction parameter: R02 has no external projection; this value still contributes to inherited floor thickness"
equation "UpperDeckHeight = 145 mm" comment "Small jars only; verify cabinet swing"
equation "FootSize = 16 mm" comment "Support foot footprint"
equation "PegSize = 8 mm" comment "Square locating peg"
equation "PegHeight = 1.5 mm" comment "Foot locating peg, not a locking fastener"
equation "FitClearance = 0.25 mm" comment "Per-side foot fit allowance; test first"
equation "BaseX = 50 mm" comment "Model datum offset"
equation "BaseY = 50 mm" comment "Model datum offset"
equation "d38 = FootHeight"
equation "d40 = ( BaseX + TowerFrame + TowerClearance ) + ( 0 mm )"
equation "d41 = ( BaseY ) + ( 0 mm )"
equation "d42 = TowerWidth - 2 * ( TowerFrame + TowerClearance )"
equation "d43 = Depth"
equation "d44 = PanHeight"
equation "d48 = ( BaseX + TowerFrame + TowerClearance ) + ( Wall )"
equation "d50 = -( -( ( FootHeight ) + FloorMin + DrainExtension * tan(DrainSlope) + ( ( Depth ) - ( Wall ) ) * tan(DrainSlope) ) )"
equation "d51 = ( ( BaseY ) + ( Wall ) )"
equation "d52 = -( -( ( FootHeight ) + FloorMin + DrainExtension * tan(DrainSlope) + ( ( Depth ) - ( ( Depth ) - Wall ) ) * tan(DrainSlope) ) )"
equation "d53 = ( ( BaseY ) + ( ( Depth ) - Wall ) )"
equation "d54 = -( -( ( FootHeight ) + PanHeight + 1 mm ) )"
equation "d55 = ( TowerWidth - 2 * ( TowerFrame + TowerClearance ) ) - 2 * Wall"
equation "d57 = ( BaseX + TowerFrame + TowerClearance ) + ( ( TowerWidth - 2 * ( TowerFrame + TowerClearance ) - 31 mm ) - DrainWidth / 2 - Wall )"
equation "d59 = -( -( FootHeight ) )"
equation "d60 = ( ( BaseY ) + ( ( Depth ) - Wall ) )"
equation "d61 = ( ( BaseY ) + ( ( Depth ) + DrainExtension ) )"
equation "d62 = -( -( ( FootHeight ) + FloorMin + DrainExtension * tan(DrainSlope) + ( ( Depth ) - ( ( Depth ) + DrainExtension ) ) * tan(DrainSlope) ) )"
equation "d63 = -( -( ( FootHeight ) + FloorMin + DrainExtension * tan(DrainSlope) + ( ( Depth ) - ( ( Depth ) - Wall ) ) * tan(DrainSlope) ) )"
equation "d64 = DrainWidth + 2 * Wall"
equation "d66 = ( BaseX + TowerFrame + TowerClearance ) + ( ( TowerWidth - 2 * ( TowerFrame + TowerClearance ) - 31 mm ) - DrainWidth / 2 - Wall )"
equation "d68 = -( -( FootHeight ) )"
equation "d69 = ( ( BaseY ) + ( ( Depth ) - Wall ) )"
equation "d70 = ( ( BaseY ) + ( ( Depth ) + DrainExtension ) )"
equation "d71 = -( -( ( ( FootHeight ) + FloorMin + DrainExtension * tan(DrainSlope) + ( ( Depth ) - ( ( Depth ) + DrainExtension ) ) * tan(DrainSlope) ) + ( 6 mm ) ) )"
equation "d72 = -( -( ( ( FootHeight ) + FloorMin + DrainExtension * tan(DrainSlope) + ( ( Depth ) - ( ( Depth ) - Wall ) ) * tan(DrainSlope) ) + ( 6 mm ) ) )"
equation "d73 = Wall"
equation "d75 = ( BaseX + TowerFrame + TowerClearance ) + ( ( TowerWidth - 2 * ( TowerFrame + TowerClearance ) - 31 mm ) + DrainWidth / 2 )"
equation "d77 = -( -( FootHeight ) )"
equation "d78 = ( ( BaseY ) + ( ( Depth ) - Wall ) )"
equation "d79 = ( ( BaseY ) + ( ( Depth ) + DrainExtension ) )"
equation "d80 = -( -( ( ( FootHeight ) + FloorMin + DrainExtension * tan(DrainSlope) + ( ( Depth ) - ( ( Depth ) + DrainExtension ) ) * tan(DrainSlope) ) + ( 6 mm ) ) )"
equation "d81 = -( -( ( ( FootHeight ) + FloorMin + DrainExtension * tan(DrainSlope) + ( ( Depth ) - ( ( Depth ) - Wall ) ) * tan(DrainSlope) ) + ( 6 mm ) ) )"
equation "d82 = Wall"
equation "d84 = ( BaseX + TowerFrame + TowerClearance ) + ( ( TowerWidth - 2 * ( TowerFrame + TowerClearance ) - 31 mm ) - DrainWidth / 2 )"
equation "d86 = -( -( ( FootHeight ) + FloorMin + DrainExtension * tan(DrainSlope) + ( ( Depth ) - ( ( Depth ) - Wall ) ) * tan(DrainSlope) ) )"
equation "d87 = ( ( BaseY ) + ( ( Depth ) - Wall ) )"
equation "d88 = -( -( ( FootHeight ) + FloorMin + DrainExtension * tan(DrainSlope) + ( ( Depth ) - ( ( Depth ) + DrainExtension ) ) * tan(DrainSlope) ) )"
equation "d89 = ( ( BaseY ) + ( ( Depth ) + DrainExtension ) )"
equation "d90 = -( -( ( FootHeight ) + PanHeight + 1 mm ) )"
equation "d91 = DrainWidth"
equation "d93 = FootHeight"
equation "d95 = ( BaseX + TowerFrame + TowerClearance ) + ( Wall )"
equation "d96 = ( BaseY ) + ( Wall )"
equation "d99 = PanHeight - DeckThick"
equation "d101 = FootHeight"
equation "d103 = ( BaseX + TowerFrame + TowerClearance ) + ( Wall )"
equation "d104 = ( BaseY ) + ( ( Depth ) - Wall - 12 mm )"
equation "d107 = PanHeight - DeckThick"
equation "d109 = FootHeight"
equation "d111 = ( BaseX + TowerFrame + TowerClearance ) + ( ( TowerWidth - 2 * ( TowerFrame + TowerClearance ) ) - Wall - 12 mm )"
equation "d112 = ( BaseY ) + ( Wall )"
equation "d115 = PanHeight - DeckThick"
equation "d117 = FootHeight"
equation "d119 = ( BaseX + TowerFrame + TowerClearance ) + ( ( TowerWidth - 2 * ( TowerFrame + TowerClearance ) ) - Wall - 12 mm )"
equation "d120 = ( BaseY ) + ( ( Depth ) - Wall - 12 mm )"
equation "d123 = PanHeight - DeckThick"
equation "d125 = ( BaseX + TowerFrame + TowerClearance ) + ( ( TowerWidth - 2 * ( TowerFrame + TowerClearance ) - 31 mm ) - DrainWidth / 2 - Wall )"
equation "d127 = -( -( ( FootHeight ) - ( 0.2 mm ) ) )"
equation "d128 = ( ( BaseY ) + ( ( Depth ) + DrainExtension - 2 mm ) )"
equation "d129 = ( ( BaseY ) + ( ( ( Depth ) + DrainExtension - 2 mm ) + ( 1 mm ) ) )"
equation "d130 = -( -( ( FootHeight ) + ( 0.6 mm ) ) )"
equation "d131 = DrainWidth + 2 * Wall"
equation "d133 = FootHeight"
equation "d135 = ( BaseX + TowerFrame + TowerClearance ) + ( ( 11 mm ) - PegSize / 2 - FitClearance )"
equation "d136 = ( BaseY ) + ( ( 11 mm ) - PegSize / 2 - FitClearance )"
equation "d137 = PegSize + 2 * FitClearance"
equation "d138 = PegSize + 2 * FitClearance"
equation "d139 = PegHeight + 0.3 mm"
equation "d141 = FootHeight"
equation "d143 = ( BaseX + TowerFrame + TowerClearance ) + ( ( 11 mm ) - PegSize / 2 - FitClearance )"
equation "d144 = ( BaseY ) + ( ( ( Depth ) - FrontFootInset ) - PegSize / 2 - FitClearance )"
equation "d145 = PegSize + 2 * FitClearance"
equation "d146 = PegSize + 2 * FitClearance"
equation "d147 = PegHeight + 0.3 mm"
equation "d149 = FootHeight"
equation "d151 = ( BaseX + TowerFrame + TowerClearance ) + ( ( ( TowerWidth - 2 * ( TowerFrame + TowerClearance ) ) - 11 mm ) - PegSize / 2 - FitClearance )"
equation "d152 = ( BaseY ) + ( ( 11 mm ) - PegSize / 2 - FitClearance )"
equation "d153 = PegSize + 2 * FitClearance"
equation "d154 = PegSize + 2 * FitClearance"
equation "d155 = PegHeight + 0.3 mm"
equation "d157 = FootHeight"
equation "d159 = ( BaseX + TowerFrame + TowerClearance ) + ( ( ( TowerWidth - 2 * ( TowerFrame + TowerClearance ) ) - 11 mm ) - PegSize / 2 - FitClearance )"
equation "d160 = ( BaseY ) + ( ( ( Depth ) - FrontFootInset ) - PegSize / 2 - FitClearance )"
equation "d161 = PegSize + 2 * FitClearance"
equation "d162 = PegSize + 2 * FitClearance"
equation "d163 = PegHeight + 0.3 mm"
equation "d165 = ( FootHeight ) + PanHeight - DeckThick"
equation "d167 = ( BaseX + TowerFrame + TowerClearance ) + ( Wall + DeckClearance )"
equation "d168 = ( BaseY ) + ( Wall + DeckClearance )"
equation "d169 = ( TowerWidth - 2 * ( TowerFrame + TowerClearance ) ) - 2 * ( Wall + DeckClearance )"
equation "d170 = ( Depth ) - 2 * ( Wall + DeckClearance )"
equation "d171 = DeckThick"
equation "d173 = ( FootHeight ) + PanHeight - DeckThick"
equation "d175 = ( BaseX + TowerFrame + TowerClearance ) + ( ( ( ( TowerWidth - 2 * ( TowerFrame + TowerClearance ) ) - ( 12 * SlotPitch + SlotWidth ) ) / 2 ) + ( 0 * SlotPitch ) )"
equation "d176 = ( BaseY ) + ( Wall + DeckClearance + RimBorder )"
equation "d177 = SlotWidth"
equation "d178 = ( Depth ) - 2 * ( Wall + DeckClearance + RimBorder )"
equation "d179 = DeckThick"
equation "d181 = ( FootHeight ) + PanHeight - DeckThick"
equation "d183 = ( BaseX + TowerFrame + TowerClearance ) + ( ( ( ( TowerWidth - 2 * ( TowerFrame + TowerClearance ) ) - ( 12 * SlotPitch + SlotWidth ) ) / 2 ) + ( 1 * SlotPitch ) )"
equation "d184 = ( BaseY ) + ( Wall + DeckClearance + RimBorder )"
equation "d185 = SlotWidth"
equation "d186 = ( Depth ) - 2 * ( Wall + DeckClearance + RimBorder )"
equation "d187 = DeckThick"
equation "d189 = ( FootHeight ) + PanHeight - DeckThick"
equation "d191 = ( BaseX + TowerFrame + TowerClearance ) + ( ( ( ( TowerWidth - 2 * ( TowerFrame + TowerClearance ) ) - ( 12 * SlotPitch + SlotWidth ) ) / 2 ) + ( 2 * SlotPitch ) )"
equation "d192 = ( BaseY ) + ( Wall + DeckClearance + RimBorder )"
equation "d193 = SlotWidth"
equation "d194 = ( Depth ) - 2 * ( Wall + DeckClearance + RimBorder )"
equation "d195 = DeckThick"
equation "d197 = ( FootHeight ) + PanHeight - DeckThick"
equation "d199 = ( BaseX + TowerFrame + TowerClearance ) + ( ( ( ( TowerWidth - 2 * ( TowerFrame + TowerClearance ) ) - ( 12 * SlotPitch + SlotWidth ) ) / 2 ) + ( 3 * SlotPitch ) )"
equation "d200 = ( BaseY ) + ( Wall + DeckClearance + RimBorder )"
equation "d201 = SlotWidth"
equation "d202 = ( Depth ) - 2 * ( Wall + DeckClearance + RimBorder )"
equation "d203 = DeckThick"
equation "d205 = ( FootHeight ) + PanHeight - DeckThick"
equation "d207 = ( BaseX + TowerFrame + TowerClearance ) + ( ( ( ( TowerWidth - 2 * ( TowerFrame + TowerClearance ) ) - ( 12 * SlotPitch + SlotWidth ) ) / 2 ) + ( 4 * SlotPitch ) )"
equation "d208 = ( BaseY ) + ( Wall + DeckClearance + RimBorder )"
equation "d209 = SlotWidth"
equation "d210 = ( Depth ) - 2 * ( Wall + DeckClearance + RimBorder )"
equation "d211 = DeckThick"
equation "d213 = ( FootHeight ) + PanHeight - DeckThick"
equation "d215 = ( BaseX + TowerFrame + TowerClearance ) + ( ( ( ( TowerWidth - 2 * ( TowerFrame + TowerClearance ) ) - ( 12 * SlotPitch + SlotWidth ) ) / 2 ) + ( 5 * SlotPitch ) )"
equation "d216 = ( BaseY ) + ( Wall + DeckClearance + RimBorder )"
equation "d217 = SlotWidth"
equation "d218 = ( Depth ) - 2 * ( Wall + DeckClearance + RimBorder )"
equation "d219 = DeckThick"
equation "d221 = ( FootHeight ) + PanHeight - DeckThick"
equation "d223 = ( BaseX + TowerFrame + TowerClearance ) + ( ( ( ( TowerWidth - 2 * ( TowerFrame + TowerClearance ) ) - ( 12 * SlotPitch + SlotWidth ) ) / 2 ) + ( 6 * SlotPitch ) )"
equation "d224 = ( BaseY ) + ( Wall + DeckClearance + RimBorder )"
equation "d225 = SlotWidth"
equation "d226 = ( Depth ) - 2 * ( Wall + DeckClearance + RimBorder )"
equation "d227 = DeckThick"
equation "d229 = ( FootHeight ) + PanHeight - DeckThick"
equation "d231 = ( BaseX + TowerFrame + TowerClearance ) + ( ( ( ( TowerWidth - 2 * ( TowerFrame + TowerClearance ) ) - ( 12 * SlotPitch + SlotWidth ) ) / 2 ) + ( 7 * SlotPitch ) )"
equation "d232 = ( BaseY ) + ( Wall + DeckClearance + RimBorder )"
equation "d233 = SlotWidth"
equation "d234 = ( Depth ) - 2 * ( Wall + DeckClearance + RimBorder )"
equation "d235 = DeckThick"
equation "d237 = ( FootHeight ) + PanHeight - DeckThick"
equation "d239 = ( BaseX + TowerFrame + TowerClearance ) + ( ( ( ( TowerWidth - 2 * ( TowerFrame + TowerClearance ) ) - ( 12 * SlotPitch + SlotWidth ) ) / 2 ) + ( 8 * SlotPitch ) )"
equation "d240 = ( BaseY ) + ( Wall + DeckClearance + RimBorder )"
equation "d241 = SlotWidth"
equation "d242 = ( Depth ) - 2 * ( Wall + DeckClearance + RimBorder )"
equation "d243 = DeckThick"
equation "d245 = ( FootHeight ) + PanHeight - DeckThick"
equation "d247 = ( BaseX + TowerFrame + TowerClearance ) + ( ( ( ( TowerWidth - 2 * ( TowerFrame + TowerClearance ) ) - ( 12 * SlotPitch + SlotWidth ) ) / 2 ) + ( 9 * SlotPitch ) )"
equation "d248 = ( BaseY ) + ( Wall + DeckClearance + RimBorder )"
equation "d249 = SlotWidth"
equation "d250 = ( Depth ) - 2 * ( Wall + DeckClearance + RimBorder )"
equation "d251 = DeckThick"
equation "d253 = ( FootHeight ) + PanHeight - DeckThick"
equation "d255 = ( BaseX + TowerFrame + TowerClearance ) + ( ( ( ( TowerWidth - 2 * ( TowerFrame + TowerClearance ) ) - ( 12 * SlotPitch + SlotWidth ) ) / 2 ) + ( 10 * SlotPitch ) )"
equation "d256 = ( BaseY ) + ( Wall + DeckClearance + RimBorder )"
equation "d257 = SlotWidth"
equation "d258 = ( Depth ) - 2 * ( Wall + DeckClearance + RimBorder )"
equation "d259 = DeckThick"
equation "d261 = ( FootHeight ) + PanHeight - DeckThick"
equation "d263 = ( BaseX + TowerFrame + TowerClearance ) + ( ( ( ( TowerWidth - 2 * ( TowerFrame + TowerClearance ) ) - ( 12 * SlotPitch + SlotWidth ) ) / 2 ) + ( 11 * SlotPitch ) )"
equation "d264 = ( BaseY ) + ( Wall + DeckClearance + RimBorder )"
equation "d265 = SlotWidth"
equation "d266 = ( Depth ) - 2 * ( Wall + DeckClearance + RimBorder )"
equation "d267 = DeckThick"
equation "d269 = ( FootHeight ) + PanHeight - DeckThick"
equation "d271 = ( BaseX + TowerFrame + TowerClearance ) + ( ( ( ( TowerWidth - 2 * ( TowerFrame + TowerClearance ) ) - ( 12 * SlotPitch + SlotWidth ) ) / 2 ) + ( 12 * SlotPitch ) )"
equation "d272 = ( BaseY ) + ( Wall + DeckClearance + RimBorder )"
equation "d273 = SlotWidth"
equation "d274 = ( Depth ) - 2 * ( Wall + DeckClearance + RimBorder )"
equation "d275 = DeckThick"
equation "d277 = ( FootHeight ) + PanHeight - DeckThick"
equation "d279 = ( BaseX + TowerFrame + TowerClearance ) + ( ( TowerWidth - 2 * ( TowerFrame + TowerClearance ) ) / 2 - 8 mm )"
equation "d280 = ( BaseY ) + ( ( Depth ) - Wall - DeckClearance - 4 mm )"
equation "d283 = DeckThick"
equation "d287 = ( BaseX + TowerFrame + TowerClearance ) + ( ( 11 mm ) - FootSize / 2 )"
equation "d288 = ( BaseY ) + ( ( 11 mm ) - FootSize / 2 )"
equation "d289 = FootSize"
equation "d290 = FootSize"
equation "d291 = FootHeight"
equation "d293 = FootHeight"
equation "d295 = ( BaseX + TowerFrame + TowerClearance ) + ( ( 11 mm ) - PegSize / 2 )"
equation "d296 = ( BaseY ) + ( ( 11 mm ) - PegSize / 2 )"
equation "d297 = PegSize"
equation "d298 = PegSize"
equation "d299 = PegHeight"
equation "d303 = ( BaseX + TowerFrame + TowerClearance ) + ( ( 11 mm ) - FootSize / 2 )"
equation "d304 = ( BaseY ) + ( ( ( Depth ) - FrontFootInset ) - FootSize / 2 )"
equation "d305 = FootSize"
equation "d306 = FootSize"
equation "d307 = FootHeight"
equation "d309 = FootHeight"
equation "d311 = ( BaseX + TowerFrame + TowerClearance ) + ( ( 11 mm ) - PegSize / 2 )"
equation "d312 = ( BaseY ) + ( ( ( Depth ) - FrontFootInset ) - PegSize / 2 )"
equation "d313 = PegSize"
equation "d314 = PegSize"
equation "d315 = PegHeight"
equation "d319 = ( BaseX + TowerFrame + TowerClearance ) + ( ( ( TowerWidth - 2 * ( TowerFrame + TowerClearance ) ) - 11 mm ) - FootSize / 2 )"
equation "d320 = ( BaseY ) + ( ( 11 mm ) - FootSize / 2 )"
equation "d321 = FootSize"
equation "d322 = FootSize"
equation "d323 = FootHeight"
equation "d325 = FootHeight"
equation "d327 = ( BaseX + TowerFrame + TowerClearance ) + ( ( ( TowerWidth - 2 * ( TowerFrame + TowerClearance ) ) - 11 mm ) - PegSize / 2 )"
equation "d328 = ( BaseY ) + ( ( 11 mm ) - PegSize / 2 )"
equation "d329 = PegSize"
equation "d330 = PegSize"
equation "d331 = PegHeight"
equation "d335 = ( BaseX + TowerFrame + TowerClearance ) + ( ( ( TowerWidth - 2 * ( TowerFrame + TowerClearance ) ) - 11 mm ) - FootSize / 2 )"
equation "d336 = ( BaseY ) + ( ( ( Depth ) - FrontFootInset ) - FootSize / 2 )"
equation "d337 = FootSize"
equation "d338 = FootSize"
equation "d339 = FootHeight"
equation "d341 = FootHeight"
equation "d343 = ( BaseX + TowerFrame + TowerClearance ) + ( ( ( TowerWidth - 2 * ( TowerFrame + TowerClearance ) ) - 11 mm ) - PegSize / 2 )"
equation "d344 = ( BaseY ) + ( ( ( Depth ) - FrontFootInset ) - PegSize / 2 )"
equation "d345 = PegSize"
equation "d346 = PegSize"
equation "d347 = PegHeight"
equation "d349 = FootHeight"
equation "d351 = ( BaseX + TowerWidth + ModuleGap ) + ( 0 mm )"
equation "d352 = ( BaseY ) + ( 0 mm )"
equation "d353 = LeftRun - TowerWidth - ModuleGap"
equation "d354 = Depth"
equation "d355 = PanHeight"
equation "d359 = ( BaseX + TowerWidth + ModuleGap ) + ( Wall )"
equation "d361 = -( -( ( FootHeight ) + FloorMin + DrainExtension * tan(DrainSlope) + ( ( Depth ) - ( Wall ) ) * tan(DrainSlope) ) )"
equation "d362 = ( ( BaseY ) + ( Wall ) )"
equation "d363 = -( -( ( FootHeight ) + FloorMin + DrainExtension * tan(DrainSlope) + ( ( Depth ) - ( ( Depth ) - Wall ) ) * tan(DrainSlope) ) )"
equation "d364 = ( ( BaseY ) + ( ( Depth ) - Wall ) )"
equation "d365 = -( -( ( FootHeight ) + PanHeight + 1 mm ) )"
equation "d366 = ( LeftRun - TowerWidth - ModuleGap ) - 2 * Wall"
equation "d368 = ( BaseX + TowerWidth + ModuleGap ) + ( ( ( LeftRun - TowerWidth - ModuleGap ) / 2 ) - DrainWidth / 2 - Wall )"
equation "d370 = -( -( FootHeight ) )"
equation "d371 = ( ( BaseY ) + ( ( Depth ) - Wall ) )"
equation "d372 = ( ( BaseY ) + ( ( Depth ) + DrainExtension ) )"
equation "d373 = -( -( ( FootHeight ) + FloorMin + DrainExtension * tan(DrainSlope) + ( ( Depth ) - ( ( Depth ) + DrainExtension ) ) * tan(DrainSlope) ) )"
equation "d374 = -( -( ( FootHeight ) + FloorMin + DrainExtension * tan(DrainSlope) + ( ( Depth ) - ( ( Depth ) - Wall ) ) * tan(DrainSlope) ) )"
equation "d375 = DrainWidth + 2 * Wall"
equation "d377 = ( BaseX + TowerWidth + ModuleGap ) + ( ( ( LeftRun - TowerWidth - ModuleGap ) / 2 ) - DrainWidth / 2 - Wall )"
equation "d379 = -( -( FootHeight ) )"
equation "d380 = ( ( BaseY ) + ( ( Depth ) - Wall ) )"
equation "d381 = ( ( BaseY ) + ( ( Depth ) + DrainExtension ) )"
equation "d382 = -( -( ( ( FootHeight ) + FloorMin + DrainExtension * tan(DrainSlope) + ( ( Depth ) - ( ( Depth ) + DrainExtension ) ) * tan(DrainSlope) ) + ( 6 mm ) ) )"
equation "d383 = -( -( ( ( FootHeight ) + FloorMin + DrainExtension * tan(DrainSlope) + ( ( Depth ) - ( ( Depth ) - Wall ) ) * tan(DrainSlope) ) + ( 6 mm ) ) )"
equation "d384 = Wall"
equation "d386 = ( BaseX + TowerWidth + ModuleGap ) + ( ( ( LeftRun - TowerWidth - ModuleGap ) / 2 ) + DrainWidth / 2 )"
equation "d388 = -( -( FootHeight ) )"
equation "d389 = ( ( BaseY ) + ( ( Depth ) - Wall ) )"
equation "d390 = ( ( BaseY ) + ( ( Depth ) + DrainExtension ) )"
equation "d391 = -( -( ( ( FootHeight ) + FloorMin + DrainExtension * tan(DrainSlope) + ( ( Depth ) - ( ( Depth ) + DrainExtension ) ) * tan(DrainSlope) ) + ( 6 mm ) ) )"
equation "d392 = -( -( ( ( FootHeight ) + FloorMin + DrainExtension * tan(DrainSlope) + ( ( Depth ) - ( ( Depth ) - Wall ) ) * tan(DrainSlope) ) + ( 6 mm ) ) )"
equation "d393 = Wall"